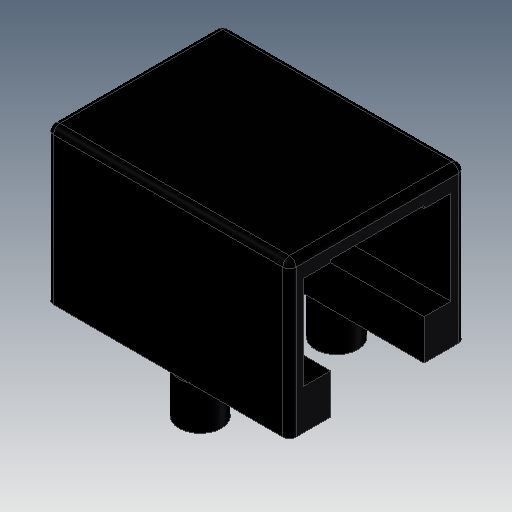
# Autodesk Inventor part: RJ12 Connector
Saved by Autodesk Inventor 2020 (Build 240168000, 168)
## iProperties
Created: 2021-02-16
Part Number: RJ12 Connector
Material: Generic
Document SubType Name: Modeling
Designer: ferrerx
Density: 1 g/cm^3
Appearance: Glossy - Black
Author: ferrerx
Autodesk Inventor part; units mm, degrees
ref_plane "YZ Plane" through (0, 0, 0) normal (1, 0, 0) x (0, 1, 0)
ref_plane "XZ Plane" through (0, 0, 0) normal (0, 1, 0) x (-1, 0, 0)
ref_plane "XY Plane" through (0, 0, 0) normal (0, 0, 1) x (1, 0, 0)
sketch "Sketch1" plane through (0, 0, 0) normal (0, 1, 0) x (-1, 0, 0)
  line L0 (0, 0) -> (18.15, 0)
  line L1 (18.15, 0) -> (18.15, -13.15)
  line L2 (18.15, -13.15) -> (0, -13.15)
  line L3 (0, -13.15) -> (0, 0)
  dimension "d0" = 18.15
  dimension "d1" = 13.15
  constraints: 8 end point, 2 parallel, 1 horizontal, 1 perpendicular
  measures "d0" distance of L1.end L2.end
  measures "d1" distance of L2.end L0.start
extrude "Extrusion1" add sketch "Sketch1" along normal blind 11.5
sketch "Sketch2" plane through (0, 0, 0) normal (0, -1, 0) x (1, 0, 0)
  circle A0 centre (-8.15, -1.475) radius 1.6
  line L0 (0, 0) -> (0, -13.15) projected
  line L1 (-18.15, -13.15) -> (-18.15, 0) projected
  line L2 (0, 0) -> (0, -13.15) projected
  line L3 (0, -6.575) -> (-18.15, -6.575) construction
  circle A1 centre (-8.15, -11.675) radius 1.6
  dimension "d5" = 10
  dimension "d6" = 3.2
  dimension "d7" = 5.1
  constraints: 2 centre point, 2 end point, 2 midpoint, 1 symmetric about line, 1 other
  measures "d5" distance from line of L1 A0.centre
  measures "d6" diameter of A0
  measures "d7" distance from line of L3 A0.centre
extrude "Extrusion2" add sketch "Sketch2" along normal blind 3.2
sketch "Sketch3" plane through (0, 0, 0) normal (1, 0, 0) x (0, 0, -1)
  line L0 (0, 0) -> (13.15, 0) projected
  line L1 (6.575, 0) -> (6.575, 11.5) construction
  line L2 (13.15, 11.5) -> (0, 11.5) projected
  line L3 (3.075, 0) -> (3.075, 3)
  line L4 (3.075, 3) -> (1.075, 3)
  line L5 (1.075, 3) -> (1.075, 10)
  line L6 (1.075, 10) -> (3.075, 10)
  line L7 (3.075, 10) -> (3.075, 10.2)
  line L8 (3.075, 10.2) -> (6.575, 10.2)
  line L9 (3.075, 0) -> (6.575, 0)
  line L10 (10.075, 0) -> (10.075, 3)
  line L11 (10.075, 3) -> (12.075, 3)
  line L12 (12.075, 3) -> (12.075, 10)
  line L13 (12.075, 10) -> (10.075, 10)
  line L14 (10.075, 10) -> (10.075, 10.2)
  line L15 (10.075, 10.2) -> (6.575, 10.2)
  line L16 (10.075, 0) -> (6.575, 0)
  dimension "d10" = 3.5
  dimension "d11" = 3
  dimension "d12" = 7
  dimension "d13" = 2
  dimension "d15" = 1.3
  constraints: 30 end point, 6 point on line, 6 symmetric about line, 4 perpendicular, 2 midpoint, 1 collinear, 1 vertical
  measures "d10" distance between parallel lines of L1 L3
  measures "d11" distance of L3.start L3.end
  measures "d12" distance of L4.end L5.end
  measures "d13" distance of L5.end L6.end
  measures "d15" distance between parallel lines of L2 L8
extrude "Extrusion3" cut sketch "Sketch3" against normal blind 13
fillet "Fillet1" radius 0.5 8 edges at (0, 5.75, -13.15) (-9.075, 11.5, -13.15) (0, 11.5, -6.575) (0, 5.75, 0) (-9.075, 11.5, 0) (-18.15, 5.75, 0) (-18.15, 11.5, -6.575) (-18.15, 5.75, -13.15)
body "Solid1"
